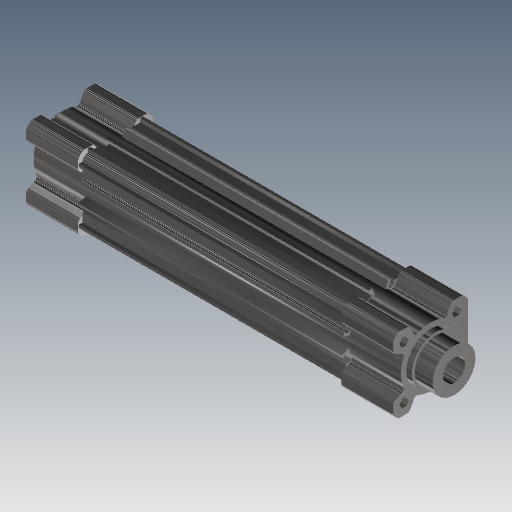
# Autodesk Inventor part: CP96S40-160(0)_BODY
Saved by Autodesk Inventor 2021 (Build 250183000, 183)
## iProperties
Part Number: CP96S40-160(0)_BODY
Material: Stainless Steel, Polished
Catalog Web Link: www.cadenas.de
Description: CP96 BODY-ISO Cylinder:Standard Double Acting,Single/Double Rod
Vendor: SMC
Document SubType Name: Modeling
Designer: partserver
Manufacturer: SMC
Mass: 2842.3 g
Surface Area: 1204.9 cm^2
Volume: 355.287 cm^3
Density: 8 g/cm^3
Appearance: Stainless - Polished
Category: PARTsolutions
Company: SMC
PSOL_IDENT_0: {$CADENAS_DATA\23d-libs\smc_jp\actuator\standard_air_cylinder\cp96_c96\cp96\parts\cp96_body.prj},201
PSOL_IDENT_1: {VTYP=3D},{NB=CP96S40-160(0)_BODY},{LINA=CP96S40-160_BODY},{NN=CP96 BODY},{DATE=18.06.2021 10:30:56
PSOL_IDENT_2: },{GEOMDATE=28.11.2018 06:56:23},{VERSION=},{LINEID=20},{WBVAR=STROKE,ROD,THREAD},{WBNUMERIC=STROKE}
PSOL_IDENT_3: {NB=CP96S40-160(0)_BODY},{LINA=CP96S40-160_BODY},{KT=DUMMY},{BORE=40},{STROKE=160},{ROD=},{THREAD=
PSOL_IDENT_4: 0},{ORDER=CP96S40-160},{A=24},{B=35},{D=16},{EE=G 1/4},{EEE=NPT 1/4},{EEND=13.157},{EED=13},{PL=14.0
PSOL_IDENT_5: },{RT=M6x1},{RTRA=6},{RTRP=1.00},{L12=6.5},{KK=M12x1.25},{SW=13},{G=37.5},{BG=16},{L8=105},{VD=4},{V
PSOL_IDENT_6: A=4},{WA=5.0},{WB=9.0},{WH=30},{ZZ=163},{ZY=213},{E=54},{R=38.0},{L2=17},{L9=4},{H=54},{LC1=6.0},{LC
PSOL_IDENT_7: 2=31.0},{RC1=2.0},{RC2=3.3},{RC3=7.0},{RC4=8.8},{RC5=3.9},{DC1=43.0},{DC2=45.0},{DC4=31.0},{HC=6.0},
PSOL_IDENT_8: {C1=53.0},{C2=47.5},{C3=36.0},{C4=40.0},{C5=20.5},{C6=23.0},{C7=21.8},{C9=21.5},{FONT=5},{SIZE=12}
NB: CP96S40-160(0)_BODY
NN: CP96 BODY
NT: ISO Cylinder:Standard Double Acting,Single/Double Rod
NBSYN: $ORDER.($THREAD.)_BODY
LINA: CP96S40-160_BODY
CATALOG: SMC (JP
BORE: 40
STROKE: 160
ROD: (-) Single rod
THREAD: on
A: 24
B: 35
D: 16
EE: G 1/4
EEE: NPT 1/4
PL: 14
RT: M6x1
L12: 6.5
KK: M12x1.25
SW: 13
G: 37.5
BG: 16
L8: 105
VD: 4
VA: 4
WA: 5
WB: 9
WH: 30
ZZ: 163
ZY: 213
E: 54
R: 38
L2: 17
L9: 4
H: 54
SUPPLIER: SMC
ARTICLENO: CP96S40-160(0)_BODY
BOMINFO: CP96S40-160_BODY
CREATOR: CADENAS GmbH
Title: CP96S40-160_BODY
Author: Cadenas PARTsolutions
Comments: ISO Cylinder:Standard Double Acting,Single/Double Rod
Autodesk Inventor part; units mm, degrees
sketch "Sketch_5" plane through (0, 0, 0) normal (1, 0, 0) x (0, 1, 0)
  line L0 (21.8566, 27) -> (17.3137, 27)
  arc A0 (17.3137, 27) -> (14.4021, 25.2532) centre (17.3137, 23.7) ccw
  line L1 (14.4021, 25.2532) -> (12.8239, 22.2947)
  arc A1 (12.8239, 22.2947) -> (12.2013, 20.6664) centre (19, 19) ccw
  arc A2 (9.3857, 19.3432) -> (12.2013, 20.6664) centre (10.2588, 21.1426) ccw
  arc A3 (9.3857, 19.3432) -> (-9.3857, 19.3432) centre (0, 0) ccw
  arc A4 (-12.2013, 20.6664) -> (-9.3857, 19.3432) centre (-10.2588, 21.1426) ccw
  arc A5 (-12.2013, 20.6664) -> (-12.8239, 22.2947) centre (-19, 19) ccw
  line L2 (-12.8239, 22.2947) -> (-14.4021, 25.2532)
  arc A6 (-14.4021, 25.2532) -> (-17.3137, 27) centre (-17.3137, 23.7) ccw
  line L3 (-17.3137, 27) -> (-21.8566, 27)
  arc A7 (-21.8566, 27) -> (-23.5705, 26.52) centre (-21.8566, 23.7) ccw
  arc A8 (-23.5705, 26.52) -> (-26.52, 23.5705) centre (-19, 19) ccw
  arc A9 (-26.52, 23.5705) -> (-27, 21.8566) centre (-23.7, 21.8566) ccw
  line L4 (-27, 21.8566) -> (-27, 17.3137)
  arc A10 (-27, 17.3137) -> (-25.2532, 14.4021) centre (-23.7, 17.3137) ccw
  line L5 (-25.2532, 14.4021) -> (-22.2947, 12.8239)
  arc A11 (-22.2947, 12.8239) -> (-20.6664, 12.2013) centre (-19, 19) ccw
  arc A12 (-19.3432, 9.3857) -> (-20.6664, 12.2013) centre (-21.1426, 10.2588) ccw
  arc A13 (-19.3432, 9.3857) -> (-19.3432, -9.3857) centre (0, 0) ccw
  arc A14 (-20.6664, -12.2013) -> (-19.3432, -9.3857) centre (-21.1426, -10.2588) ccw
  arc A15 (-20.6664, -12.2013) -> (-22.2947, -12.8239) centre (-19, -19) ccw
  line L6 (-22.2947, -12.8239) -> (-25.2532, -14.4021)
  arc A16 (-25.2532, -14.4021) -> (-27, -17.3137) centre (-23.7, -17.3137) ccw
  line L7 (-27, -17.3137) -> (-27, -21.8566)
  arc A17 (-27, -21.8566) -> (-26.52, -23.5705) centre (-23.7, -21.8566) ccw
  arc A18 (-26.52, -23.5705) -> (-23.5705, -26.52) centre (-19, -19) ccw
  arc A19 (-23.5705, -26.52) -> (-21.8566, -27) centre (-21.8566, -23.7) ccw
  line L8 (-21.8566, -27) -> (-17.3137, -27)
  arc A20 (-17.3137, -27) -> (-14.4021, -25.2532) centre (-17.3137, -23.7) ccw
  line L9 (-14.4021, -25.2532) -> (-12.8239, -22.2947)
  arc A21 (-12.8239, -22.2947) -> (-12.2013, -20.6664) centre (-19, -19) ccw
  arc A22 (-9.3857, -19.3432) -> (-12.2013, -20.6664) centre (-10.2588, -21.1426) ccw
  arc A23 (-9.3857, -19.3432) -> (9.3857, -19.3432) centre (0, 0) ccw
  arc A24 (12.2013, -20.6664) -> (9.3857, -19.3432) centre (10.2588, -21.1426) ccw
  arc A25 (12.2013, -20.6664) -> (12.8239, -22.2947) centre (19, -19) ccw
  line L10 (12.8239, -22.2947) -> (14.4021, -25.2532)
  arc A26 (14.4021, -25.2532) -> (17.3137, -27) centre (17.3137, -23.7) ccw
  line L11 (17.3137, -27) -> (21.8566, -27)
  arc A27 (21.8566, -27) -> (23.5705, -26.52) centre (21.8566, -23.7) ccw
  arc A28 (23.5705, -26.52) -> (26.52, -23.5705) centre (19, -19) ccw
  arc A29 (26.52, -23.5705) -> (27, -21.8566) centre (23.7, -21.8566) ccw
  line L12 (27, -21.8566) -> (27, -17.3137)
  arc A30 (27, -17.3137) -> (25.2532, -14.4021) centre (23.7, -17.3137) ccw
  line L13 (25.2532, -14.4021) -> (22.2947, -12.8239)
  arc A31 (22.2947, -12.8239) -> (20.6664, -12.2013) centre (19, -19) ccw
  arc A32 (19.3432, -9.3857) -> (20.6664, -12.2013) centre (21.1426, -10.2588) ccw
  arc A33 (19.3432, -9.3857) -> (19.3432, 9.3857) centre (0, 0) ccw
  arc A34 (20.6664, 12.2013) -> (19.3432, 9.3857) centre (21.1426, 10.2588) ccw
  arc A35 (20.6664, 12.2013) -> (22.2947, 12.8239) centre (19, 19) ccw
  line L14 (22.2947, 12.8239) -> (25.2532, 14.4021)
  arc A36 (25.2532, 14.4021) -> (27, 17.3137) centre (23.7, 17.3137) ccw
  line L15 (27, 17.3137) -> (27, 21.8566)
  arc A37 (27, 21.8566) -> (26.52, 23.5705) centre (23.7, 21.8566) ccw
  arc A38 (26.52, 23.5705) -> (23.5705, 26.52) centre (19, 19) ccw
  arc A39 (23.5705, 26.52) -> (21.8566, 27) centre (21.8566, 23.7) ccw
  constraints: 80 point on circle, 40 centre point, 32 end point
extrude "Extrusion1" add sketch "Sketch_5" along normal blind 37.5
sketch "Sketch_29" plane through (37.5, 0, 0) normal (1, 0, 0) x (0, 0, -1)
  line L0 (-26.6665, 4.6322) -> (-21.3373, 2.6397)
  arc A0 (-21.3373, 2.6397) -> (-20.9239, -4.9436) centre (0, 0) ccw
  line L1 (-20.9239, -4.9436) -> (-25.6487, -6.9492)
  line L2 (-25.6487, -6.9492) -> (-24.8184, -8.9052)
  line L3 (-24.8184, -8.9052) -> (-23.9947, -8.5556)
  arc A1 (-22.8225, -11.3171) -> (-23.9947, -8.5556) centre (-22.0231, -9.3482) ccw
  line L4 (-22.8225, -11.3171) -> (-23.75, -11.7108)
  line L5 (-23.75, -11.7108) -> (-23.75, -18)
  line L6 (-23.75, -18) -> (-26.5, -18)
  line L7 (-26.5, -18) -> (-26.5, -20)
  line L8 (-26.5, -20) -> (-23.75, -20)
  arc A2 (-23.75, -20) -> (-20, -23.75) centre (-20, -20) ccw
  line L9 (-20, -23.75) -> (-20, -26.5)
  line L10 (-20, -26.5) -> (-18, -26.5)
  line L11 (-18, -26.5) -> (-18, -23.75)
  line L12 (-18, -23.75) -> (-11.7089, -23.75)
  line L13 (-11.7089, -23.75) -> (-11.3424, -22.7698)
  line L14 (-11.3424, -22.7698) -> (-11.9513, -22.5421)
  line L15 (-11.9513, -22.5421) -> (-10.7255, -19.2638)
  line L16 (-10.7255, -19.2638) -> (-4.5435, -21.5751)
  line L17 (-4.5435, -21.5751) -> (-5.7692, -24.8535)
  line L18 (-5.7692, -24.8535) -> (-6.3781, -24.6259)
  line L19 (-6.3781, -24.6259) -> (-6.8333, -25.8435)
  line L20 (-6.8333, -25.8435) -> (-4.6322, -26.6665)
  line L21 (-4.6322, -26.6665) -> (-2.6397, -21.3373)
  arc A3 (-2.6397, -21.3373) -> (4.9436, -20.9239) centre (0, 0) ccw
  line L22 (4.9436, -20.9239) -> (6.9492, -25.6487)
  line L23 (6.9492, -25.6487) -> (8.9052, -24.8184)
  line L24 (8.9052, -24.8184) -> (8.5556, -23.9947)
  arc A4 (11.3171, -22.8225) -> (8.5556, -23.9947) centre (9.3482, -22.0231) ccw
  line L25 (11.3171, -22.8225) -> (11.7108, -23.75)
  line L26 (11.7108, -23.75) -> (18, -23.75)
  line L27 (18, -23.75) -> (18, -26.5)
  line L28 (18, -26.5) -> (20, -26.5)
  line L29 (20, -26.5) -> (20, -23.75)
  arc A5 (20, -23.75) -> (23.75, -20) centre (20, -20) ccw
  line L30 (23.75, -20) -> (26.5, -20)
  line L31 (26.5, -20) -> (26.5, -18)
  line L32 (26.5, -18) -> (23.75, -18)
  line L33 (23.75, -18) -> (23.75, -11.7089)
  line L34 (23.75, -11.7089) -> (22.7698, -11.3424)
  line L35 (22.7698, -11.3424) -> (22.5421, -11.9513)
  line L36 (22.5421, -11.9513) -> (19.2638, -10.7255)
  line L37 (19.2638, -10.7255) -> (21.5751, -4.5435)
  line L38 (21.5751, -4.5435) -> (24.8535, -5.7692)
  line L39 (24.8535, -5.7692) -> (24.6259, -6.3781)
  line L40 (24.6259, -6.3781) -> (25.8435, -6.8333)
  line L41 (25.8435, -6.8333) -> (26.6665, -4.6322)
  line L42 (26.6665, -4.6322) -> (21.3373, -2.6397)
  arc A6 (21.3373, -2.6397) -> (20.9239, 4.9436) centre (0, 0) ccw
  line L43 (20.9239, 4.9436) -> (25.6487, 6.9492)
  line L44 (25.6487, 6.9492) -> (24.8184, 8.9052)
  line L45 (24.8184, 8.9052) -> (23.9947, 8.5556)
  arc A7 (22.8225, 11.3171) -> (23.9947, 8.5556) centre (22.0231, 9.3482) ccw
  line L46 (22.8225, 11.3171) -> (23.75, 11.7108)
  line L47 (23.75, 11.7108) -> (23.75, 18)
  line L48 (23.75, 18) -> (26.5, 18)
  line L49 (26.5, 18) -> (26.5, 20)
  line L50 (26.5, 20) -> (23.75, 20)
  arc A8 (23.75, 20) -> (20, 23.75) centre (20, 20) ccw
  line L51 (20, 23.75) -> (20, 26.5)
  line L52 (20, 26.5) -> (18, 26.5)
  line L53 (18, 26.5) -> (18, 23.75)
  line L54 (18, 23.75) -> (11.7089, 23.75)
  line L55 (11.7089, 23.75) -> (11.3424, 22.7698)
  line L56 (11.3424, 22.7698) -> (11.9513, 22.5421)
  line L57 (11.9513, 22.5421) -> (10.7255, 19.2638)
  line L58 (10.7255, 19.2638) -> (4.5435, 21.5751)
  line L59 (4.5435, 21.5751) -> (5.7692, 24.8535)
  line L60 (5.7692, 24.8535) -> (6.3781, 24.6259)
  line L61 (6.3781, 24.6259) -> (6.8333, 25.8435)
  line L62 (6.8333, 25.8435) -> (4.6322, 26.6665)
  line L63 (4.6322, 26.6665) -> (2.6397, 21.3373)
  arc A9 (2.6397, 21.3373) -> (-4.9436, 20.9239) centre (0, 0) ccw
  line L64 (-4.9436, 20.9239) -> (-6.9492, 25.6487)
  line L65 (-6.9492, 25.6487) -> (-8.9052, 24.8184)
  line L66 (-8.9052, 24.8184) -> (-8.5556, 23.9947)
  arc A10 (-11.3171, 22.8225) -> (-8.5556, 23.9947) centre (-9.3482, 22.0231) ccw
  line L67 (-11.3171, 22.8225) -> (-11.7108, 23.75)
  line L68 (-11.7108, 23.75) -> (-18, 23.75)
  line L69 (-18, 23.75) -> (-18, 26.5)
  line L70 (-18, 26.5) -> (-20, 26.5)
  line L71 (-20, 26.5) -> (-20, 23.75)
  arc A11 (-20, 23.75) -> (-23.75, 20) centre (-20, 20) ccw
  line L72 (-23.75, 20) -> (-26.5, 20)
  line L73 (-26.5, 20) -> (-26.5, 18)
  line L74 (-26.5, 18) -> (-23.75, 18)
  line L75 (-23.75, 18) -> (-23.75, 11.7089)
  line L76 (-23.75, 11.7089) -> (-22.7698, 11.3424)
  line L77 (-22.7698, 11.3424) -> (-22.5421, 11.9513)
  line L78 (-22.5421, 11.9513) -> (-19.2638, 10.7255)
  line L79 (-19.2638, 10.7255) -> (-21.5751, 4.5435)
  line L80 (-21.5751, 4.5435) -> (-24.8535, 5.7692)
  line L81 (-24.8535, 5.7692) -> (-24.6259, 6.3781)
  line L82 (-24.6259, 6.3781) -> (-25.8435, 6.8333)
  line L83 (-25.8435, 6.8333) -> (-26.6665, 4.6322)
  constraints: 168 end point, 24 point on circle, 12 centre point
extrude "Extrusion2" add sketch "Sketch_29" along normal blind 190
sketch "Sketch_36" plane through (0, 27, 0) normal (0, 1, 0) x (1, 0, 0)
  line L0 (0, -6) -> (18, -6)
  arc A0 (18, -6) -> (25, 1) centre (18, 1) ccw
  arc A1 (26, 2) -> (25, 1) centre (26, 1) ccw
  line L1 (26, 2) -> (37.5, 2)
  line L2 (37.5, 2) -> (37.5, 19)
  line L3 (37.5, 19) -> (0, 19)
  line L4 (0, 19) -> (0, -6)
  constraints: 10 end point, 4 point on circle, 2 centre point
extrude "Extrusion3" add sketch "Sketch_36" against normal blind 13
sketch "Sketch_35" plane through (265, 0, 0) normal (1, 0, 0) x (0, 0, -1)
  line L0 (-27, 21.8566) -> (-27, 17.3137)
  arc A0 (-27, 17.3137) -> (-25.2532, 14.4021) centre (-23.7, 17.3137) ccw
  line L1 (-25.2532, 14.4021) -> (-22.2947, 12.8239)
  arc A1 (-22.2947, 12.8239) -> (-20.6664, 12.2013) centre (-19, 19) ccw
  arc A2 (-19.3432, 9.3857) -> (-20.6664, 12.2013) centre (-21.1426, 10.2588) ccw
  arc A3 (-19.3432, 9.3857) -> (-19.3432, -9.3857) centre (0, 0) ccw
  arc A4 (-20.6664, -12.2013) -> (-19.3432, -9.3857) centre (-21.1426, -10.2588) ccw
  arc A5 (-20.6664, -12.2013) -> (-22.2947, -12.8239) centre (-19, -19) ccw
  line L2 (-22.2947, -12.8239) -> (-25.2532, -14.4021)
  arc A6 (-25.2532, -14.4021) -> (-27, -17.3137) centre (-23.7, -17.3137) ccw
  line L3 (-27, -17.3137) -> (-27, -21.8566)
  arc A7 (-27, -21.8566) -> (-26.52, -23.5705) centre (-23.7, -21.8566) ccw
  arc A8 (-26.52, -23.5705) -> (-23.5705, -26.52) centre (-19, -19) ccw
  arc A9 (-23.5705, -26.52) -> (-21.8566, -27) centre (-21.8566, -23.7) ccw
  line L4 (-21.8566, -27) -> (-17.3137, -27)
  arc A10 (-17.3137, -27) -> (-14.4021, -25.2532) centre (-17.3137, -23.7) ccw
  line L5 (-14.4021, -25.2532) -> (-12.8239, -22.2947)
  arc A11 (-12.8239, -22.2947) -> (-12.2013, -20.6664) centre (-19, -19) ccw
  arc A12 (-9.3857, -19.3432) -> (-12.2013, -20.6664) centre (-10.2588, -21.1426) ccw
  arc A13 (-9.3857, -19.3432) -> (9.3857, -19.3432) centre (0, 0) ccw
  arc A14 (12.2013, -20.6664) -> (9.3857, -19.3432) centre (10.2588, -21.1426) ccw
  arc A15 (12.2013, -20.6664) -> (12.8239, -22.2947) centre (19, -19) ccw
  line L6 (12.8239, -22.2947) -> (14.4021, -25.2532)
  arc A16 (14.4021, -25.2532) -> (17.3137, -27) centre (17.3137, -23.7) ccw
  line L7 (17.3137, -27) -> (21.8566, -27)
  arc A17 (21.8566, -27) -> (23.5705, -26.52) centre (21.8566, -23.7) ccw
  arc A18 (23.5705, -26.52) -> (26.52, -23.5705) centre (19, -19) ccw
  arc A19 (26.52, -23.5705) -> (27, -21.8566) centre (23.7, -21.8566) ccw
  line L8 (27, -21.8566) -> (27, -17.3137)
  arc A20 (27, -17.3137) -> (25.2532, -14.4021) centre (23.7, -17.3137) ccw
  line L9 (25.2532, -14.4021) -> (22.2947, -12.8239)
  arc A21 (22.2947, -12.8239) -> (20.6664, -12.2013) centre (19, -19) ccw
  arc A22 (19.3432, -9.3857) -> (20.6664, -12.2013) centre (21.1426, -10.2588) ccw
  arc A23 (19.3432, -9.3857) -> (19.3432, 9.3857) centre (0, 0) ccw
  arc A24 (20.6664, 12.2013) -> (19.3432, 9.3857) centre (21.1426, 10.2588) ccw
  arc A25 (20.6664, 12.2013) -> (22.2947, 12.8239) centre (19, 19) ccw
  line L10 (22.2947, 12.8239) -> (25.2532, 14.4021)
  arc A26 (25.2532, 14.4021) -> (27, 17.3137) centre (23.7, 17.3137) ccw
  line L11 (27, 17.3137) -> (27, 21.8566)
  arc A27 (27, 21.8566) -> (26.52, 23.5705) centre (23.7, 21.8566) ccw
  arc A28 (26.52, 23.5705) -> (23.5705, 26.52) centre (19, 19) ccw
  arc A29 (23.5705, 26.52) -> (21.8566, 27) centre (21.8566, 23.7) ccw
  line L12 (21.8566, 27) -> (17.3137, 27)
  arc A30 (17.3137, 27) -> (14.4021, 25.2532) centre (17.3137, 23.7) ccw
  line L13 (14.4021, 25.2532) -> (12.8239, 22.2947)
  arc A31 (12.8239, 22.2947) -> (12.2013, 20.6664) centre (19, 19) ccw
  arc A32 (9.3857, 19.3432) -> (12.2013, 20.6664) centre (10.2588, 21.1426) ccw
  arc A33 (9.3857, 19.3432) -> (-9.3857, 19.3432) centre (0, 0) ccw
  arc A34 (-12.2013, 20.6664) -> (-9.3857, 19.3432) centre (-10.2588, 21.1426) ccw
  arc A35 (-12.2013, 20.6664) -> (-12.8239, 22.2947) centre (-19, 19) ccw
  line L14 (-12.8239, 22.2947) -> (-14.4021, 25.2532)
  arc A36 (-14.4021, 25.2532) -> (-17.3137, 27) centre (-17.3137, 23.7) ccw
  line L15 (-17.3137, 27) -> (-21.8566, 27)
  arc A37 (-21.8566, 27) -> (-23.5705, 26.52) centre (-21.8566, 23.7) ccw
  arc A38 (-23.5705, 26.52) -> (-26.52, 23.5705) centre (-19, 19) ccw
  arc A39 (-26.52, 23.5705) -> (-27, 21.8566) centre (-23.7, 21.8566) ccw
  constraints: 80 point on circle, 40 centre point, 32 end point
extrude "Extrusion4" add sketch "Sketch_35" against normal blind 37.5
sketch "Sketch_38" plane through (0, 27, 0) normal (0, 1, 0) x (1, 0, 0)
  line L0 (227.5, -2) -> (227.5, -19)
  line L1 (227.5, -19) -> (265, -19)
  line L2 (265, -19) -> (265, 6)
  line L3 (265, 6) -> (247, 6)
  arc A0 (247, 6) -> (240, -1) centre (247, -1) ccw
  arc A1 (239, -2) -> (240, -1) centre (239, -1) ccw
  line L4 (239, -2) -> (227.5, -2)
  constraints: 10 end point, 4 point on circle, 2 centre point
extrude "Extrusion5" add sketch "Sketch_38" against normal blind 13
sketch "Sketch_1" plane through (0, 0, 0) normal (0, 0, 1) x (1, 0, 0)
  line L0 (0, 0) -> (-17, 0)
  line L1 (-17, 0) -> (-17, 15.5)
  line L2 (-17, 15.5) -> (-4, 15.5)
  line L3 (-4, 15.5) -> (-4, 17.5)
  line L4 (-4, 17.5) -> (0, 17.5)
  line L5 (0, 17.5) -> (0, 0)
  line L6 (0, 0) -> (-17, 0)
  constraints: 14 end point
revolve "Revolution1" add sketch "Sketch_1" angle 360 about axis through (0, 0, 0) along (1, 0, 0)
sketch "Sketch_2" plane through (0, 0, 0) normal (0, 0, 1) x (1, 0, 0)
  line L0 (269, 0) -> (265, 0)
  line L1 (265, 0) -> (265, 17.5)
  line L2 (265, 17.5) -> (269, 17.5)
  line L3 (269, 17.5) -> (269, 0)
  line L4 (269, 0) -> (265, 0)
  constraints: 10 end point
revolve "Revolution2" add sketch "Sketch_2" angle 360 about axis through (269, 0, 0) along (1, 0, 0)
sketch "Sketch_3" plane through (0, 0, 0) normal (0, 0, 1) x (1, 0, 0)
  line L0 (207.5, 0) -> (-17, 0)
  line L1 (-17, 0) -> (-17, 8)
  line L2 (-17, 8) -> (37.5, 8)
  line L3 (37.5, 8) -> (37.5, 20)
  line L4 (37.5, 20) -> (207.5, 20)
  line L5 (207.5, 20) -> (207.5, 0)
  line L6 (207.5, 0) -> (-17, 0)
  constraints: 14 end point
revolve "Revolution3" cut sketch "Sketch_3" angle 360 about axis through (207.5, 0, 0) along (1, 0, 0)
sketch "Sketch_25" plane through (0, 0, -19) normal (0, 0, 1) x (1, 0, 0)
  line L0 (17.4194, 19) -> (0, 19)
  line L1 (0, 19) -> (0, 21)
  line L2 (0, 21) -> (4, 21)
  line L3 (4, 21) -> (4, 22)
  line L4 (4, 22) -> (4.5415, 21.4585)
  line L5 (4.5415, 21.4585) -> (16, 21.4585)
  line L6 (16, 21.4585) -> (17.4194, 19)
  line L7 (17.4194, 19) -> (0, 19)
  constraints: 16 end point
revolve "Revolution4" cut sketch "Sketch_25" angle 360 about axis through (17.4194, 19, -19) along (1, 0, 0)
thread "Thread1" size "M6x1" class "6H" standard "ISO Metric profile" full length
pattern_linear "Rectangular Pattern1" count 2 spacing 38 along (0, 0, 1) count 2 spacing 38 along (0, -1, 0) of "Revolution4"
sketch "Sketch_6" plane through (0, 0, 0) normal (1, 0, 0) x (0, 1, 0)
  line L0 (17.2679, -16) -> (15.5359, -19)
  line L1 (15.5359, -19) -> (17.2679, -22)
  line L2 (17.2679, -22) -> (20.7321, -22)
  line L3 (20.7321, -22) -> (22.4641, -19)
  line L4 (22.4641, -19) -> (20.7321, -16)
  line L5 (20.7321, -16) -> (17.2679, -16)
  constraints: 12 end point
extrude "Extrusion6" cut sketch "Sketch_6" along normal blind 4
pattern_linear "Rectangular Pattern2" count 2 spacing 38 along (0, 0, 1) count 2 spacing 38 along (0, -1, 0) of "Extrusion6"
sketch "Sketch_26" plane through (0, 0, -19) normal (0, 0, 1) x (1, 0, 0)
  line L0 (265, 19) -> (247.5806, 19)
  line L1 (247.5806, 19) -> (249, 21.4585)
  line L2 (249, 21.4585) -> (260.4585, 21.4585)
  line L3 (260.4585, 21.4585) -> (261, 22)
  line L4 (261, 22) -> (261, 21)
  line L5 (261, 21) -> (265, 21)
  line L6 (265, 21) -> (265, 19)
  line L7 (265, 19) -> (247.5806, 19)
  constraints: 16 end point
revolve "Revolution5" cut sketch "Sketch_26" angle 360 about axis through (265, 19, -19) along (1, 0, 0)
thread "Thread2" size "M6x1" class "6H" standard "ISO Metric profile" full length
pattern_linear "Rectangular Pattern3" count 2 spacing 38 along (0, 0, 1) count 2 spacing 38 along (0, -1, 0) of "Revolution5"
sketch "Sketch_12" plane through (265, 0, 0) normal (1, 0, 0) x (0, 0, -1)
  line L0 (16, 17.2679) -> (19, 15.5359)
  line L1 (19, 15.5359) -> (22, 17.2679)
  line L2 (22, 17.2679) -> (22, 20.7321)
  line L3 (22, 20.7321) -> (19, 22.4641)
  line L4 (19, 22.4641) -> (16, 20.7321)
  line L5 (16, 20.7321) -> (16, 17.2679)
  constraints: 12 end point
extrude "Extrusion7" cut sketch "Sketch_12" against normal blind 4
pattern_linear "Rectangular Pattern4" count 2 spacing 38 along (0, 0, 1) count 2 spacing 38 along (0, -1, 0) of "Extrusion7"
sketch "Sketch_20" plane through (14, 0, 0) normal (1, 0, 0) x (0, 0, -1)
  line L0 (5, 10.6961) -> (5, 27)
  line L1 (5, 27) -> (11.5785, 27)
  line L2 (11.5785, 27) -> (10.7225, 26.144)
  line L3 (10.7225, 26.144) -> (10.7225, 14)
  line L4 (10.7225, 14) -> (5, 10.6961)
  line L5 (5, 10.6961) -> (5, 27)
  constraints: 12 end point
revolve "Revolution6" cut sketch "Sketch_20" angle 360 about axis through (14, 10.6961, -5) along (0, -1, 0)
thread "Thread3" size "G13.157x1.337" designation "G 1/4" standard "ISO Pipe Threads" full length
sketch "Sketch_21" plane through (0, 0, -9) normal (0, 0, 1) x (1, 0, 0)
  line L0 (31, 22) -> (31, 27)
  line L1 (31, 27) -> (34.9, 27)
  line L2 (34.9, 27) -> (34.9, 22)
  line L3 (34.9, 22) -> (31, 22)
  line L4 (31, 22) -> (31, 27)
  constraints: 10 end point
revolve "Revolution7" cut sketch "Sketch_21" angle 360 about axis through (31, 22, -9) along (0, -1, 0)
sketch "Sketch_23" plane through (251, 0, 0) normal (1, 0, 0) x (0, 0, -1)
  line L0 (-5, 10.6961) -> (-5, 27)
  line L1 (-5, 27) -> (1.5785, 27)
  line L2 (1.5785, 27) -> (0.7225, 26.144)
  line L3 (0.7225, 26.144) -> (0.7225, 14)
  line L4 (0.7225, 14) -> (-5, 10.6961)
  line L5 (-5, 10.6961) -> (-5, 27)
  constraints: 12 end point
revolve "Revolution8" cut sketch "Sketch_23" angle 360 about axis through (251, 10.6961, 5) along (0, -1, 0)
thread "Thread4" size "G13.157x1.337" designation "G 1/4" standard "ISO Pipe Threads" full length
sketch "Sketch_24" plane through (0, 0, 9) normal (0, 0, 1) x (1, 0, 0)
  line L0 (234, 22) -> (234, 27)
  line L1 (234, 27) -> (237.9, 27)
  line L2 (237.9, 27) -> (237.9, 22)
  line L3 (237.9, 22) -> (234, 22)
  line L4 (234, 22) -> (234, 27)
  constraints: 10 end point
revolve "Revolution9" cut sketch "Sketch_24" angle 360 about axis through (234, 22, 9) along (0, -1, 0)
ref_plane "BODY_BL_XY" through (0, 0, 0) normal (-1, 0, 0) x (0, 0, -1)
ref_plane "BODY_BL_YZ" through (0, 0, 0) normal (0, 0, -1) x (0, -1, 0)
ref_plane "BODY_BL_ZX" through (0, 0, 0) normal (0, -1, 0) x (-1, 0, 0)
ref_plane "BODY_BL1_XY" through (265, 0, 0) normal (1, 0, 0) x (0, 0, -1)
ref_plane "BODY_BL1_YZ" through (265, 0, 0) normal (0, 0, -1) x (0, 1, 0)
ref_plane "BODY_BL1_ZX" through (265, 0, 0) normal (0, 1, 0) x (1, 0, 0)
ref_plane "BODY_BR_XY" through (0, 0, 0) normal (-1, 0, 0) x (0, 0, -1)
ref_plane "BODY_BR_YZ" through (0, 0, 0) normal (0, 0, -1) x (0, -1, 0)
ref_plane "BODY_BR_ZX" through (0, 0, 0) normal (0, -1, 0) x (-1, 0, 0)
ref_plane "BODY_BR1_XY" through (265, 0, 0) normal (1, 0, 0) x (0, 0, -1)
ref_plane "BODY_BR1_YZ" through (265, 0, 0) normal (0, 0, -1) x (0, 1, 0)
ref_plane "BODY_BR1_ZX" through (265, 0, 0) normal (0, 1, 0) x (1, 0, 0)
ref_plane "BODY_DUMMY_XY" through (0, 0, 0) normal (-1, 0, 0) x (0, 0, -1)
ref_plane "BODY_DUMMY_YZ" through (0, 0, 0) normal (0, 0, -1) x (0, -1, 0)
ref_plane "BODY_DUMMY_ZX" through (0, 0, 0) normal (0, -1, 0) x (-1, 0, 0)
ref_plane "BODY_MOUNT1_XY" through (0, 0, 0) normal (-1, 0, 0) x (0, 0, -1)
ref_plane "BODY_MOUNT1_YZ" through (0, 0, 0) normal (0, 0, -1) x (0, -1, 0)
ref_plane "BODY_MOUNT1_ZX" through (0, 0, 0) normal (0, -1, 0) x (-1, 0, 0)
ref_plane "BODY_MOUNT2_XY" through (265, 0, 0) normal (1, 0, 0) x (0, 0, -1)
ref_plane "BODY_MOUNT2_YZ" through (265, 0, 0) normal (0, 0, -1) x (0, 1, 0)
ref_plane "BODY_MOUNT2_ZX" through (265, 0, 0) normal (0, 1, 0) x (1, 0, 0)
ref_plane "BODY_ROD_XY" through (0, 0, 0) normal (1, 0, 0) x (0, 0, -1)
ref_plane "BODY_ROD_YZ" through (0, 0, 0) normal (0, 0, -1) x (0, 1, 0)
ref_plane "BODY_ROD_ZX" through (0, 0, 0) normal (0, 1, 0) x (1, 0, 0)
ref_plane "BODY_SWA1_XY" through (37.5, 22.0231, 9.3482) normal (-1, 0, 0) x (0, 0.3907311, -0.9205049)
ref_plane "BODY_SWA1_YZ" through (37.5, 22.0231, 9.3482) normal (0, 0.3907311, -0.9205049) x (0, -0.9205049, -0.3907311)
ref_plane "BODY_SWA1_ZX" through (37.5, 22.0231, 9.3482) normal (0, -0.9205049, -0.3907311) x (-1, 0, 0)
ref_plane "BODY_SWB1_XY" through (227.5, -9.3482, 22.0231) normal (1, 0, 0) x (0, 0.3907311, -0.9205049)
ref_plane "BODY_SWB1_YZ" through (227.5, -9.3482, 22.0231) normal (0, 0.3907311, -0.9205049) x (0, 0.9205049, 0.3907311)
ref_plane "BODY_SWB1_ZX" through (227.5, -9.3482, 22.0231) normal (0, 0.9205049, 0.3907311) x (1, 0, 0)
ref_plane "G3_XY" through (227.5, 0, 0) normal (0, 1, 0) x (1, 0, 0)
ref_plane "G3_YZ" through (227.5, 0, 0) normal (1, 0, 0) x (0, 0, -1)
ref_plane "G3_ZX" through (227.5, 0, 0) normal (0, 0, -1) x (0, 1, 0)
ref_plane "G4_XY" through (265, 0, 0) normal (0, 1, 0) x (1, 0, 0)
ref_plane "G4_YZ" through (265, 0, 0) normal (1, 0, 0) x (0, 0, -1)
ref_plane "G4_ZX" through (265, 0, 0) normal (0, 0, -1) x (0, 1, 0)
ref_plane "R4_XY" through (0, 19, -19) normal (1, 0, 0) x (0, 0, -1)
ref_plane "R4_YZ" through (0, 19, -19) normal (0, 0, -1) x (0, 1, 0)
ref_plane "R4_ZX" through (0, 19, -19) normal (0, 1, 0) x (1, 0, 0)
ref_plane "VA2_XY" through (269, 0, 0) normal (0, 1, 0) x (1, 0, 0)
ref_plane "VA2_YZ" through (269, 0, 0) normal (1, 0, 0) x (0, 0, -1)
ref_plane "VA2_ZX" through (269, 0, 0) normal (0, 0, -1) x (0, 1, 0)
ref_plane "WA2_XY" through (14, 27, 0) normal (0, 1, 0) x (1, 0, 0)
ref_plane "WA2_YZ" through (14, 27, 0) normal (1, 0, 0) x (0, 0, -1)
ref_plane "WA2_ZX" through (14, 27, 0) normal (0, 0, -1) x (0, 1, 0)
body "Solid1"
